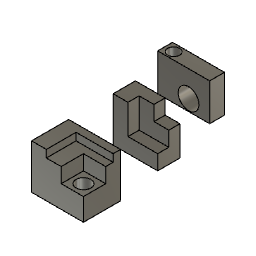
1.2.4 (Autodesk Fusion 360 design; units mm, degrees)
Autodesk Fusion 360 part; units mm, degrees
box "BoxPrimitive1" add length 63.5 width 88.9 height 25.4 placed x (0, 0, -1) y (-1, 0, 0) z (0, 1, 0) at (50.8, 0, 50.8) makes body 1
move_body "Move1" bodies 1 to x (1, 0, 0) y (0, 1, 0) z (0, 0, 1) at (0, 0, 12.7)
hole "Hole1" at (-23.1269, 12.456, 63.5) direction (0, 0, -1) diameter 20.32 depth 86.36 tip angle 180 bodies 1
hole "Hole2" at (14.7308, 0, 19.1582) direction (0, 1, 0) diameter 35.56 depth 33.02 tip angle 180 bodies 1
box "BoxPrimitive2" add length 38.1 width 76.2 height 25.4 placed x (0, -1, 0) y (1, 0, 0) z (0, 0, 1) at (0, -76.2, 0) separate body makes body 2
box "BoxPrimitive3" add length 19.05 width 76.2 height 50.8 placed x (0, -1, 0) y (1, 0, 0) z (0, 0, 1) at (0, -76.2, 25.4) bodies 2
box "BoxPrimitive4" add length 19.05 width 25.4 height 50.8 placed x (0, -1, 0) y (1, 0, 0) z (0, 0, 1) at (0, -95.25, 25.4) bodies 2
box "BoxPrimitive5" cut length 25.4 width 25.4 height -20.32 placed x (0, 0, -1) y (1, 0, 0) z (0, -1, 0) at (50.8, -95.25, 76.2) bodies 2
box "BoxPrimitive6" add length 63.5 width 88.9 height 38.1 placed x (0, -1, 0) y (1, 0, 0) z (0, 0, 1) at (0, -190.5, 0) separate body makes body 3
box "BoxPrimitive7" add length 63.5 width 50.8 height 25.4 placed x (0, 1, 0) y (-1, 0, 0) z (0, 0, 1) at (50.8, -254, 38.1) bodies 3
box "BoxPrimitive8" add length 25.4 width 38.1 height 25.4 placed x (0, -1, 0) y (1, 0, 0) z (0, 0, 1) at (50.8, -190.5, 38.1) bodies 3
box "BoxPrimitive9" add length 63.5 width 25.4 height 12.7 placed x (0, 1, 0) y (-1, 0, 0) z (0, 0, 1) at (25.4, -254, 63.5) bodies 3
box "BoxPrimitive10" add length 12.7 width 63.5 height 12.7 placed x (0, -1, 0) y (1, 0, 0) z (0, 0, 1) at (25.4, -190.5, 63.5) bodies 3
hole "Hole3" at (69.85, -234.95, 38.1) direction (0, 0, -1) diameter 25.4 depth 50.8 tip angle 118 bodies 3
copy_body "Body->Comp1" bodies 3 removing the originals makes body 4 in component "Component"
copy_body "Body->Comp2" bodies 2 removing the originals makes body 5 in component "Component'"
copy_body "Body->Comp3" bodies 1 removing the originals makes body 6 in component "Shape1"
component "Component" placed x (1, 0, 0) y (0, 1, 0) z (0, 0, 1) at (0, 0, 0)
component "Component'" placed x (1, 0, 0) y (0, 1, 0) z (0, 0, 1) at (0, 0, 0)
component "Shape1" placed x (1, 0, 0) y (0, 1, 0) z (0, 0, 1) at (0, 0, 0)
named bodies: "Shape1"
